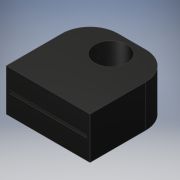
# Autodesk Inventor part: AUfsatz
Saved by Autodesk Inventor 2019 (Build 230136000, 136)
## iProperties
Created: 2020-04-12
Part Number: AUfsatz
Material: ABS Plastic
Document SubType Name: Modeling
Designer: Erle
Mass: 0.756099 g
Surface Area: 7.5072 cm^2
Volume: 0.713301 cm^3
Density: 1.06 g/cm^3
Appearance: Glossy - Black
Author: Erle
Autodesk Inventor part; units mm, degrees
ref_plane "YZ Plane" through (0, 0, 0) normal (1, 0, 0) x (0, 1, 0)
ref_plane "XZ Plane" through (0, 0, 0) normal (0, 1, 0) x (-1, 0, 0)
ref_plane "XY Plane" through (0, 0, 0) normal (0, 0, 1) x (1, 0, 0)
sketch "Sketch1" plane through (0, 0, 0) normal (0, 1, 0) x (-1, 0, 0)
  line L0 (6, 0) -> (-6, 0)
  line L1 (-6, 0) -> (-6, -12)
  line L2 (-6, -12) -> (6, -12)
  line L3 (6, -12) -> (6, 0)
  point P0 (0, 0)
  point P1 (0, 0)
  dimension "d0" = 12
  dimension "d1" = 12
  constraints: 8 end point, 2 parallel, 1 coincident, 1 horizontal, 1 horizontal alignment, 1 midpoint, 1 perpendicular
  measures "d0" distance of L0.end L1.end
  measures "d1" distance of L1.end L2.end
extrude "Extrusion1" add sketch "Sketch1" along normal blind 6
sketch "Sketch2" plane through (0, 6, 0) normal (0, 1, 0) x (1, 0, 0)
  line L0 (6, 12) -> (-6, 12) projected
  line L1 (-6, 0) -> (6, 0) projected
  point P0 (0, 0)
  point P1 (0, 9)
  point P2 (0, 0)
  dimension "d4" = 3
  constraints: 1 midpoint, 1 vertical alignment
  measures "d4" distance from line of L0 point (0, 9)
hole "Hole1" at (0, 6, -9) direction (0, -1, 0) diameter 4.6 depth 5
fillet "Fillet1" radius 4 2 edges at (-6, 3, -12) (6, 3, -12)
sketch "Sketch3" plane through (-6, 0, 0) normal (0, 0, 1) x (1, 0, 0)
  line L0 (0.5, 2.8) -> (11.5, 2.8)
  line L1 (11.5, 2.8) -> (11.5, 3.2)
  line L2 (11.5, 3.2) -> (0.5, 3.2)
  line L3 (0.5, 3.2) -> (0.5, 2.8)
  line L4 (0, 0) -> (12, 0) projected
  line L5 (0, 0) -> (0, 6) projected
  point P0 (6, 0)
  point P1 (6, 2.8)
  point P2 (6, 0)
  point P3 (0.5, 3)
  point P4 (0, 3)
  dimension "d13" = 0.4
  dimension "d14" = 11
  constraints: 8 end point, 4 midpoint, 2 parallel, 1 horizontal, 1 horizontal alignment, 1 perpendicular, 1 vertical alignment
  measures "d13" distance of L0.end L1.end
  measures "d14" distance of L1.end L2.end
extrude "Extrusion2" cut sketch "Sketch3" against normal blind 6
body "Solid1"
